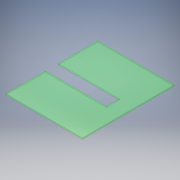
# Autodesk Inventor part: paddle collection ramp
Saved by Autodesk Inventor 2019 (Build 230136000, 136)
## iProperties
Created: 2018-11-13
Part Number: paddle collection ramp
Material: Generic
Document SubType Name: Modeling
Designer: User
Density: 1 g/cm^3
Appearance: Polycarbonate - Clear(1)
Author: User
Autodesk Inventor part; units mm, degrees
ref_plane "YZ Plane" through (0, 0, 0) normal (1, 0, 0) x (0, 1, 0)
ref_plane "XZ Plane" through (0, 0, 0) normal (0, 1, 0) x (-1, 0, 0)
ref_plane "XY Plane" through (0, 0, 0) normal (0, 0, 1) x (1, 0, 0)
sketch "Sketch1" plane through (0, 0, 0) normal (0, 1, 0) x (-1, 0, 0)
  line L0 (0, 0) -> (127, 0)
  line L1 (127, 0) -> (127, -152.4)
  line L2 (127, -152.4) -> (0, -152.4)
  line L3 (0, -152.4) -> (0, 0)
  line L4 (127, -65.405) -> (25.4, -65.405)
  line L5 (25.4, -65.405) -> (25.4, -86.995)
  line L6 (25.4, -86.995) -> (127, -86.995)
  line L7 (127, -86.995) -> (127, -65.405)
  dimension "d0" = 152.4
  dimension "d1" = 127
  dimension "d2" = 21.59
  dimension "d3" = 65.405
  dimension "d4" = 101.6
  constraints: 16 end point, 4 parallel, 2 horizontal, 2 perpendicular, 1 point on line
  measures "d0" distance of L0.end L1.end
  measures "d1" distance of L1.end L2.end
  measures "d2" distance between parallel lines of L6 L4
  measures "d3" distance between parallel lines of L2 L6
  measures "d4" distance of L4.start L4.end
extrude "Extrusion1" add sketch "Sketch1" along normal blind 1.8542 contours L0 L1 L4 L5 L6 L2 L3
equation "\"d3\" = -0.5 * d2 + 0.5 * d0"
body "Solid1"
